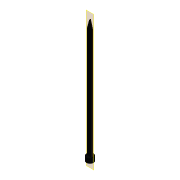
# Autodesk Inventor part: Zip tie start
Saved by Autodesk Inventor 2015 SP1 (Build 190203100, 203)
## iProperties
Created: 2015-04-17
Part Number: Zip tie start
Material: Generic
Document SubType Name: Modeling
Designer: datenney
Density: 1 g/cm^3
Appearance: Smooth - Black
Author: datenney
Autodesk Inventor part; units mm, degrees
ref_plane "YZ Plane" through (0, 0, 0) normal (1, 0, 0) x (0, 1, 0)
sketch "Sketch1" plane through (0, 0, 0) normal (0, 0, 1) x (1, 0, 0)
  line L0 (-1.905, -50.8) -> (1.905, -50.8)
  line L1 (1.905, -50.8) -> (1.905, 50.8)
  line L2 (1.905, 50.8) -> (-1.905, 50.8) construction
  line L3 (-1.905, 50.8) -> (-1.905, -50.8)
  line L4 (-1.905, -50.8) -> (1.905, 50.8) construction
  line L5 (1.905, -50.8) -> (-1.905, 50.8) construction
  line L6 (-1.905, 50.8) -> (0, 57.8088)
  line L7 (0, 57.8088) -> (1.905, 50.8)
  line L8 (0, 50.8) -> (0, 57.8088) construction
  point P0 (0, 0)
  dimension "d0" = 3.81
  dimension "d1" = 101.6
  constraints: 18 end point, 3 midpoint, 2 parallel, 1 horizontal, 1 perpendicular, 1 vertical
  measures "d0" distance of L0.start L0.end
  measures "d1" distance of L1.end L0.end
extrude "Extrusion1" add sketch "Sketch1" along normal blind 1.397
sketch "Sketch2" plane through (-1.905, -50.8, 0) normal (0, -1, 0) x (1, 0, 0)
  line L0 (0, 0) -> (3.81, 1.397) construction
  line L1 (3.81, 1.397) -> (3.81, 0) construction
  line L2 (3.81, 0) -> (0, 1.397) construction
  circle A0 centre (1.905, 0.6985) radius 3.175
  point P0 (1.905, 0)
  dimension "d4" = 6.35
  constraints: 6 end point, 1 centre point, 1 midpoint, 1 vertical
  measures "d4" diameter of A0
extrude "Extrusion2" add sketch "Sketch2" against normal blind 4.0005
ref_plane "Work Plane1" through (0, -48.7997, 0.6985) normal (0, 1, 0) x (1, 0, 0)
ref_plane "Work Plane2" through (0, -50.8, 0.6985) normal (0, -1, 0) x (1, 0, 0)
ref_plane "Work Plane3" through (0, 0, 0.6985) normal (0, 0, 1) x (1, 0, 0)
body "Solid1"
